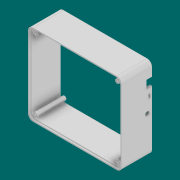
# Autodesk Inventor part: Housing
Saved by Autodesk Inventor 2020.1 (Build 241239000, 239)
## iProperties
Created: 2019-07-22
Part Number: Housing
Material: Generic
Document SubType Name: Modeling
Designer: Pluscrafter
Density: 1 g/cm^3
Appearance: Default
Author: Pluscrafter
Autodesk Inventor part; units mm, degrees
ref_plane "YZ Plane" through (0, 0, 0) normal (1, 0, 0) x (0, 1, 0)
ref_plane "XZ Plane" through (0, 0, 0) normal (0, 1, 0) x (-1, 0, 0)
ref_plane "XY Plane" through (0, 0, 0) normal (0, 0, 1) x (1, 0, 0)
sketch "Sketch1" plane through (0, 0, 0) normal (0, 0, 1) x (1, 0, 0)
  line L0 (13.2756, 161.973) -> (183.2756, 161.973)
  line L1 (193.2756, 151.973) -> (193.2756, 6.973)
  line L2 (183.2756, -3.027) -> (13.2756, -3.027)
  line L3 (3.2756, 6.973) -> (3.2756, 151.973)
  arc A0 (13.2756, 161.973) -> (3.2756, 151.973) centre (13.2756, 151.973) ccw
  arc A1 (193.2756, 151.973) -> (183.2756, 161.973) centre (183.2756, 151.973) ccw
  arc A2 (183.2756, -3.027) -> (193.2756, 6.973) centre (183.2756, 6.973) ccw
  arc A3 (3.2756, 6.973) -> (13.2756, -3.027) centre (13.2756, 6.973) ccw
  circle A4 centre (13.2756, 151.973) radius 1.5
  circle A5 centre (183.2756, 151.973) radius 1.5
  circle A6 centre (183.2756, 6.973) radius 1.5
  circle A7 centre (13.2756, 6.973) radius 1.5
  line L4 (15.2756, 159.973) -> (181.2756, 159.973)
  line L5 (191.2756, 149.973) -> (191.2756, 8.973)
  line L6 (181.2756, -1.027) -> (15.2756, -1.027)
  line L7 (5.2756, 8.973) -> (5.2756, 149.973)
  line L8 (11.2756, 163.973) -> (185.2756, 163.973)
  line L9 (195.2756, 153.973) -> (195.2756, 4.973)
  line L10 (185.2756, -5.027) -> (11.2756, -5.027)
  line L11 (1.2756, 4.973) -> (1.2756, 153.973)
  arc A8 (195.2756, 153.973) -> (185.2756, 163.973) centre (185.2756, 153.973) ccw
  arc A9 (11.2756, 163.973) -> (1.2756, 153.973) centre (11.2756, 153.973) ccw
  arc A10 (1.2756, 4.973) -> (11.2756, -5.027) centre (11.2756, 4.973) ccw
  arc A11 (185.2756, -5.027) -> (195.2756, 4.973) centre (185.2756, 4.973) ccw
  arc A12 (9.8418, 149.9214) -> (16.7094, 154.0246) centre (13.2756, 151.973) ccw
  line L12 (16.7094, 154.0246) -> (13.2761, 159.771)
  line L13 (16.7094, 154.0246) -> (9.8418, 149.9214) construction
  line L14 (9.8418, 149.9214) -> (6.7189, 155.1482)
  arc A13 (15.2756, 159.973) -> (13.2761, 159.771) centre (15.2756, 149.973) ccw
  arc A14 (6.7189, 155.1482) -> (5.2756, 149.973) centre (15.2756, 149.973) ccw
  arc A15 (181.4201, 155.5166) -> (185.7337, 148.8174) centre (183.2756, 151.973) ccw
  arc A16 (185.2426, 10.4559) -> (181.3086, 3.49) centre (183.2756, 6.973) ccw
  arc A17 (16.2722, 4.3233) -> (9.8626, 9.059) centre (13.2756, 6.973) ccw
  line L15 (185.7337, 148.8174) -> (190.8637, 152.8135)
  line L16 (185.7337, 148.8174) -> (181.4201, 155.5166) construction
  line L17 (181.4201, 155.5166) -> (186.7789, 158.3225)
  arc A18 (191.2756, 149.973) -> (190.8637, 152.8135) centre (181.2756, 149.973) ccw
  arc A19 (186.7789, 158.3225) -> (181.2756, 159.973) centre (181.2756, 149.973) ccw
  line L18 (16.2722, 4.3233) -> (12.0222, -0.483)
  line L19 (16.2722, 4.3233) -> (9.8626, 9.059) construction
  line L20 (9.8626, 9.059) -> (6.6833, 3.8571)
  arc A20 (5.2756, 8.973) -> (6.6833, 3.8571) centre (15.2756, 8.973) ccw
  arc A21 (12.0222, -0.483) -> (15.2756, -1.027) centre (15.2756, 8.973) ccw
  line L21 (185.2426, 10.4559) -> (191.1069, 7.144)
  line L22 (185.2426, 10.4559) -> (181.3086, 3.49) construction
  line L23 (181.3086, 3.49) -> (186.5944, 0.5048)
  arc A22 (181.2756, -1.027) -> (186.5944, 0.5048) centre (181.2756, 8.973) ccw
  arc A23 (191.1069, 7.144) -> (191.2756, 8.973) centre (181.2756, 8.973) ccw
  point P0 (0, 0)
  point P1 (193.2756, -3.027)
  point P2 (193.2756, 161.973)
  point P3 (3.2756, -3.027)
  point P4 (191.2756, -1.027)
  point P5 (191.2756, 159.973)
  point P6 (5.2756, -1.027)
  point P7 (195.2756, -5.027)
  point P8 (195.2756, 163.973)
  point P9 (1.2756, -5.027)
  dimension "d0" = 190
  dimension "d1" = 165
  dimension "d2" = 10
  dimension "a" = 3
  dimension "d4" = 3
  dimension "d5" = 3
  dimension "d6" = 3
  dimension "d7" = 186
  dimension "d8" = 161
  dimension "d9" = 2
  dimension "d10" = 2
  dimension "d11" = 2
  dimension "d12" = 2
  dimension "d14" = 194
  dimension "d15" = 169
  dimension "d16" = 2
  dimension "d17" = 2
  dimension "d18" = 10
  dimension "d19" = 8
  dimension "d20" = 8
  dimension "d21" = 8
  dimension "d22" = 8
  constraints: 48 end point, 40 point on circle, 32 tangent, 24 centre point, 18 point on line, 8 coincident, 6 equal radius, 6 parallel, 5 perpendicular, 3 horizontal
  measures "d0" distance of point (193.276, -3.027) point (3.276, -3.027)
  measures "d1" distance of point (193.276, 161.973) point (193.276, -3.027)
  measures "d2" radius of A0
  measures "a" diameter of A4
  measures "d4" diameter of A5
  measures "d5" diameter of A6
  measures "d6" diameter of A7
  measures "d7" distance of point (191.276, -1.027) point (5.276, -1.027)
  measures "d8" distance of point (191.276, 159.973) point (191.276, -1.027)
  measures "d9" distance between parallel lines of L2 L6
  measures "d10" distance between parallel lines of L1 L5
  measures "d11" distance between parallel lines of L3 L7
  measures "d12" distance between parallel lines of L4 L0
  measures "d14" distance of point (195.276, -5.027) point (1.276, -5.027)
  measures "d15" distance of point (195.276, 163.973) point (195.276, -5.027)
  measures "d16" distance between parallel lines of L0 L8
  measures "d17" distance between parallel lines of L1 L9
  measures "d18" radius of A8
  measures "d19" diameter of A12
  measures "d20" diameter of A15
  measures "d21" diameter of A16
  measures "d22" diameter of A17
extrude "Extrusion1" add sketch "Sketch1" along normal blind 63 contours L8 A8 L9 A11 L10 A10 L11 A9
extrude "Extrusion2" add sketch "Sketch1" along normal blind 60 contours L0 A1 L1 A2 L2 A3 L3 A0
sketch "Sketch2" plane through (195.2756, 4.973, 0) normal (1, 0, 0) x (0, 0, -1)
  line L0 (0, 0) -> (0, 149) construction
  line L1 (0, 149) -> (-63, 149) construction
  line L2 (-63, 0) -> (-63, 149) construction
  line L3 (0, 0) -> (-63, 0) construction
  line L4 (-11.4, 114.7) -> (0, 114.7)
  line L5 (0, 114.7) -> (0, 131.3)
  line L6 (0, 131.3) -> (-11.4, 131.3)
  line L7 (-11.4, 131.3) -> (-11.4, 114.7)
  line L8 (0, 0) -> (0, 149) projected
  line L9 (0, 94.8) -> (-6.8, 94.8)
  line L10 (-6.8, 94.8) -> (-6.8, 103.2)
  line L11 (-6.8, 103.2) -> (0, 103.2)
  line L12 (0, 103.2) -> (0, 94.8)
  line L13 (0, 94.8) -> (-4.4, 94.8)
  line L14 (-4.4, 94.8) -> (-4.4, 103.2)
  line L15 (-4.4, 103.2) -> (0, 103.2)
  line L16 (0, 103.2) -> (0, 94.8)
  circle A0 centre (-10, 69.8) radius 3.95
  point P0 (0, -4.973)
  dimension "d27" = 11.4
  dimension "d28" = 16.6
  dimension "d29" = 17.7
  dimension "d30" = 11.5
  dimension "d31" = 6.8
  dimension "d32" = 8.4
  dimension "d33" = 4.4
  dimension "d34" = 7.9
  dimension "d35" = 25
  dimension "d36" = 10
  constraints: 24 end point, 6 parallel, 3 horizontal, 3 perpendicular, 3 point on line, 1 centre point
  measures "d27" distance of L5.end L6.end
  measures "d28" distance of L6.end L4.start
  measures "d29" distance between parallel lines of L6 L1
  measures "d30" distance between parallel lines of L4 L11
  measures "d31" distance of L10.end L11.end
  measures "d32" distance of L9.end L10.end
  measures "d33" distance between parallel lines of L12 L14
  measures "d34" diameter of A0
  measures "d35" vertical distance of A0.centre L13.end
  measures "d36" distance from line of L0 A0.centre
extrude "Extrusion3" cut sketch "Sketch2" against normal blind 10 contours L7 L6 L5 L4 | L14 L9 L10 L11 | A0
sketch "Sketch3" plane through (1.2756, 4.973, 0) normal (-1, 0, 0) x (0, 0, 1)
  line L0 (0, 149) -> (0, 0) projected
  line L1 (0, 0) -> (63, 0) projected
  line L2 (63, 149) -> (63, 0) projected
  line L3 (0, 149) -> (63, 149) projected
  line L4 (0, 4) -> (0, 145) projected
  line L5 (0, 129) -> (10.2, 129)
  line L6 (10.2, 129) -> (10.2, 111.5)
  line L7 (10.2, 111.5) -> (0, 111.5)
  line L8 (0, 111.5) -> (0, 129)
  point P0 (0, -4.973)
  point P1 (0, 111.5)
  dimension "d39" = 17.5
  dimension "d40" = 10.2
  dimension "d41" = 20
  constraints: 8 end point, 2 parallel, 1 horizontal, 1 perpendicular, 1 point on line
  measures "d39" distance of L5.end L6.end
  measures "d40" distance of L6.end L7.end
  measures "d41" distance between parallel lines of L3 L5
extrude "Extrusion4" cut sketch "Sketch3" against normal blind 10 contours L5 L6 L7 L0
equation "\"d4\" = a"
equation "\"d5\" = a"
equation "\"d6\" = a"
body "Solid1"
